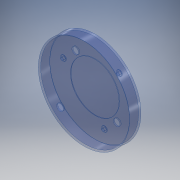
# Autodesk Inventor part: 底盘
Saved by Autodesk Inventor 2018 (Build 220112000, 112)
## iProperties
Created: 2020-11-22
Part Number: 底盘
Material: 水
Document SubType Name: Modeling
Designer: OHHHHHHHHHH
Density: 0.9983 g/cm^3
Appearance: 热带地区蓝色
Author: OHHHHHHHHHH
## iProperties of the stored document 底盘_3D 打印.ipt
Created: 2020-11-30
Part Number: 底盘_3D 打印
Material: 常规
Document SubType Name: Modeling
Designer: OHHHHHHHHHH
Density: 1 g/cm^3
Appearance: 默认
Author: OHHHHHHHHHH
Autodesk Inventor part; units mm, degrees
ref_plane "YZ Plane" through (0, 0, 0) normal (1, 0, 0) x (0, 1, 0)
ref_plane "XZ Plane" through (0, 0, 0) normal (0, 1, 0) x (-1, 0, 0)
ref_plane "XY Plane" through (0, 0, 0) normal (0, 0, 1) x (1, 0, 0)
sketch "草图1" plane through (0, 0, 0) normal (0, 1, 0) x (-1, 0, 0)
  circle A0 centre (0, 0) radius 67.5
  dimension "d0" = 135
  constraints: 1 centre point, 1 coincident
  measures "d0" diameter of A0
extrude "拉伸1" add sketch "草图1" along normal blind 17
sketch "草图3" plane through (0, 17, 0) normal (0, 1, 0) x (1, 0, 0)
  circle A0 centre (35, -35) radius 4
  point P0 (0, 0)
  dimension "d8" = 8
  dimension "d9" = 35
  dimension "d10" = 35
  constraints: 1 centre point
  measures "d8" diameter of A0
  measures "d9" horizontal distance of point (0, 0) A0.centre
  measures "d10" horizontal distance of point (0, 0) A0.centre
extrude "拉伸3" add sketch "草图3" along normal blind 1
shell "抽壳1" thickness 1.8 removed faces 1 at (33.7054, 18, 35.3191)
sketch "草图6" plane through (0, 17, 0) normal (0, 1, 0) x (1, 0, 0)
  circle A0 centre (0, 0) radius 36
  dimension "d17" = 72
  constraints: 1 centre point, 1 coincident
  measures "d17" diameter of A0
extrude "拉伸5" cut sketch "草图6" against normal blind 1
sketch "草图7" plane through (0, 0, 0) normal (0, -1, 0) x (1, 0, 0)
  circle A0 centre (-12.941, 48.2963) radius 5
  line L0 (0, 0) -> (-12.941, 48.2963)
  line L1 (-94.5, 0) -> (94.5, 0) projected
  circle A1 centre (35, 35) radius 2.2 projected
  line L2 (0, 0) -> (35, 35)
  dimension "d25" = 10
  dimension "d26" = 50
  dimension "d42" = 60
  constraints: 4 end point, 1 centre point
  measures "d25" diameter of A0
  measures "d26" distance of L0.start L0.end
  measures "d42" angle of L2 L0
extrude "拉伸6" cut sketch "草图7" against normal blind 2 contours A0
pattern_circular "环形阵列1" count 3 over 360 about axis through (0, 17, 0) along (0, -1, 0) of "拉伸3"
sketch "草图8" plane through (12.8109, 18, -47.8109) normal (0, 1, 0) x (1, 0, 0)
  circle A0 centre (0, 0) radius 2
  point P0 (-12.8109, -47.8109)
  dimension "d32" = 4
  constraints: 1 centre point
  measures "d32" diameter of A0
extrude "拉伸7" cut sketch "草图8" against normal blind 3
sketch "草图9" plane through (-47.8109, 18, 12.8109) normal (0, 1, 0) x (1, 0, 0)
  circle A0 centre (0, 0) radius 2
  point P0 (47.8109, 12.8109)
  dimension "d35" = 4
  constraints: 1 centre point
  measures "d35" diameter of A0
extrude "拉伸8" cut sketch "草图9" against normal blind 3
pattern_circular "环形阵列2" count 3 over 360 about axis through (0, 0, 0) along (0, 1, 0) of "拉伸6"
